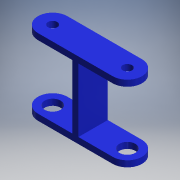
# Autodesk Inventor part: Middle_leg
Saved by Autodesk Inventor 2017 (Build 210142000, 142)
## iProperties
Part Number: Middle_leg
Material: Generic
Document SubType Name: Modeling
Designer: alex-
Appearance: Blue - Wall Paint - Glossy
Author: alex-
Autodesk Inventor part; units mm, degrees
ref_plane "YZ Plane" through (0, 0, 0) normal (1, 0, 0) x (0, 1, 0)
ref_plane "XZ Plane" through (0, 0, 0) normal (0, 1, 0) x (-1, 0, 0)
ref_plane "XY Plane" through (0, 0, 0) normal (0, 0, 1) x (1, 0, 0)
sketch "Sketch3" plane through (0, 0, 0) normal (0, 1, 0) x (-1, 0, 0)
  line L0 (2.5, 12) -> (-2.5, 12)
  line L1 (-2.5, 12) -> (-2.5, -12)
  line L2 (-2.5, -12) -> (2.5, -12)
  line L3 (2.5, -12) -> (2.5, 12)
  point P0 (0, 0)
  point P1 (0, 12)
  point P2 (2.5, 0)
  dimension "d6" = 5
  dimension "d7" = 24
  constraints: 8 end point, 2 midpoint, 2 parallel, 1 horizontal, 1 horizontal alignment, 1 perpendicular, 1 vertical alignment
  measures "d6" distance of L0.start L0.end
  measures "d7" distance of L2.end L0.start
extrude "Extrusion3" add sketch "Sketch3" along normal blind 62
sketch "Sketch4" plane through (2.5, 0, 12) normal (1, 0, 0) x (0, 0, -1)
  line L0 (0, 62) -> (24, 62)
  line L1 (24, 62) -> (24, 57)
  line L2 (24, 57) -> (0, 57)
  line L3 (0, 57) -> (0, 62)
  line L4 (0, 5) -> (24, 5)
  line L5 (24, 5) -> (24, 0)
  line L6 (24, 0) -> (0, 0)
  line L7 (0, 0) -> (0, 5)
  line L8 (0, 62) -> (24, 62) projected
  line L9 (0, 0) -> (24, 0) projected
  line L10 (0, 0) -> (0, 62) projected
  point P0 (12, 0)
  point P1 (12, 62)
  point P2 (12, 0)
  point P3 (12, 57)
  point P4 (12, 62)
  point P5 (12, 5)
  point P6 (12, 0)
  point P7 (0, 59.5)
  dimension "d10" = 5
  constraints: 16 end point, 9 midpoint, 4 parallel, 3 point on line, 2 horizontal, 2 perpendicular, 2 vertical alignment, 1 collinear
  measures "d10" distance of L0.end L1.end
extrude "Extrusion4" add sketch "Sketch4" along normal blind 40 and the other way blind 45
fillet "Fillet4" radius 12 8 edges at (42.5, 2.5, -12) (42.5, 2.5, 12) (42.5, 59.5, 12) (42.5, 59.5, -12) (-42.5, 59.5, 12) (-42.5, 2.5, 12) (-42.5, 59.5, -12) (-42.5, 2.5, -12)
sketch "Sketch8" plane through (0, 62, 0) normal (0, 1, 0) x (1, 0, 0)
  circle A0 centre (-30.5, 0) radius 3.75
  circle A1 centre (30.5, 0) radius 3.75
  arc A2 (-30.5, 12) -> (-30.5, -12) centre (-30.5, 0) ccw projected
  arc A3 (30.5, -12) -> (30.5, 12) centre (30.5, 0) ccw projected
  point P0 (0, 0)
  dimension "d27" = 7.5
  constraints: 2 centre point, 2 concentric, 1 equal radius
  measures "d27" diameter of A0
extrude "Extrusion7" cut sketch "Sketch8" against normal up to surface (5 mm away)
sketch "Sketch9" plane through (0, 0, 0) normal (0, -1, 0) x (1, 0, 0)
  circle A0 centre (-30.5, 0) radius 6.5
  circle A1 centre (30.5, 0) radius 6.5
  arc A2 (-30.5, 12) -> (-30.5, -12) centre (-30.5, 0) ccw projected
  arc A3 (30.5, -12) -> (30.5, 12) centre (30.5, 0) ccw projected
  point P0 (0, 0)
  dimension "d30" = 13
  constraints: 2 centre point, 2 concentric, 1 equal radius
  measures "d30" diameter of A0
extrude "Extrusion8" cut sketch "Sketch9" against normal up to next
equation "\"d6\" = b_mat_thickness"
equation "\"d7\" = sa_diameter"
equation "\"d10\" = b_mat_thickness"
equation "\"d24\" = d11 + b_mat_thickness"
equation "\"d26\" = 0.5 * sa_diameter"
equation "\"d30\" = bb_outer_diameter"
equation "\"b_mat_thickness\" = 5"
equation "\"sa_diameter\" = 24"
equation "\"d11\" = 40"
equation "\"bb_outer_diameter\" = 13"
body "Solid2"
